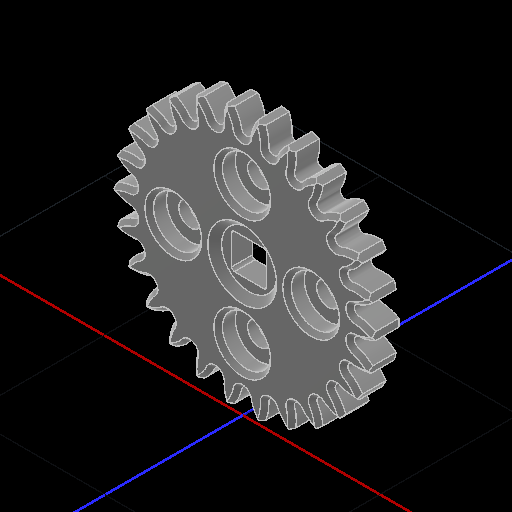
# Autodesk Inventor part: 26t
Saved by Autodesk Inventor 2025.2 (Build 292293000, 293)
## iProperties
Created: 2025-11-16
Part Number: 26t
Material: white pla
Document SubType Name: Modeling
Designer: cloudy
Density: 1 g/cm^3
Appearance: Smooth - Dark Gray
Mass: 8.30169 g
Surface Area: 51.1957 cm^2
Volume: 8.30169 cm^3
Author: cloudy
Autodesk Inventor part; units mm, degrees
ref_plane "YZ Plane" through (0, 0, 0) normal (1, 0, 0) x (0, 1, 0)
ref_plane "XZ Plane" through (0, 0, 0) normal (0, 1, 0) x (-1, 0, 0)
ref_plane "XY Plane" through (0, 0, 0) normal (0, 0, 1) x (1, 0, 0)
sketch "Sketch1" plane through (0, 0, 0) normal (0, 0, 1) x (1, 0, 0)
  spline S0 degree 3 poles (-2.1609, 23.7142) (-2.1092, 23.6364) (-2.0057, 23.4806) (-1.8586, 23.2418) (-1.7174, 22.9994) (-1.5833, 22.7529) (-1.4568, 22.5025) (-1.3387, 22.2481) (-1.2298, 21.9896) (-1.1311, 21.7269) (-1.0453, 21.4599) (-0.9712, 21.1889) (-0.9358, 20.9577) (-0.8951, 20.7751) (-0.8519, 20.6415) (-0.7979, 20.5119) (-0.7264, 20.3909) (-0.6401, 20.2798) (-0.5521, 20.2018) (-0.4739, 20.1504) (-0.4118, 20.1177) (-0.347, 20.0908) (-0.2793, 20.0718) (-0.2104, 20.0585) (-0.1169, 20.053) (0, 20.0563) (0.1169, 20.053) (0.2104, 20.0585) (0.2793, 20.0718) (0.347, 20.0908) (0.4118, 20.1177) (0.4739, 20.1504) (0.5521, 20.2018) (0.6401, 20.2798) (0.7264, 20.3909) (0.7979, 20.5119) (0.8519, 20.6415) (0.8951, 20.7751) (0.9358, 20.9577) (0.9712, 21.1889) (1.0453, 21.4599) (1.1311, 21.7269) (1.2298, 21.9896) (1.3387, 22.2481) (1.4568, 22.5025) (1.5833, 22.7529) (1.7174, 22.9994) (1.8586, 23.2418) (2.0057, 23.4806) (2.1092, 23.6364) (2.1609, 23.7142) knots 0 0 0 0 0.028048 0.056097 0.084146 0.112194 0.140242 0.16829 0.196338 0.224386 0.252432 0.280477 0.308521 0.322545 0.336563 0.350579 0.36459 0.378601 0.392611 0.399624 0.406632 0.413644 0.420653 0.427666 0.434674 0.448699 0.462724 0.469733 0.476745 0.483754 0.490767 0.497774 0.504787 0.518798 0.532808 0.546819 0.560835 0.574853 0.588877 0.616922 0.644966 0.673013 0.70106 0.729108 0.757156 0.785204 0.813253 0.841301 0.86935 0.897398 0.897398 0.897398 0.897398
  circle A0 centre (0, 0) radius 20.055 construction
  circle A1 centre (0, 0) radius 20.8847 construction
  circle A2 centre (0, 0) radius 22.225 construction
  circle A3 centre (0, 0) radius 23.8125
  point P0 (-2.0071, 23.4797)
  point P1 (-1.8596, 23.2412)
  point P2 (-1.7186, 22.9987)
  point P3 (-1.5846, 22.7523)
  point P4 (-1.4582, 22.5019)
  point P5 (-1.3402, 22.2474)
  point P6 (-1.2315, 21.9889)
  point P7 (-1.1332, 21.7262)
  point P8 (-1.0472, 21.4592)
  point P9 (-0.9765, 21.1878)
  point P10 (-0.9246, 20.9122)
  point P11 (-0.893, 20.7756)
  point P12 (-0.8501, 20.6422)
  point P13 (-0.795, 20.5133)
  point P14 (-0.7239, 20.3925)
  point P15 (-0.6369, 20.2827)
  point P16 (-0.532, 20.1899)
  point P17 (-0.4733, 20.1514)
  point P18 (-0.4114, 20.1187)
  point P19 (-0.3465, 20.0921)
  point P20 (-0.2791, 20.0727)
  point P21 (-0.2102, 20.06)
  point P22 (-0.1402, 20.0551)
  point P23 (0, 20.055)
  point P24 (0.1402, 20.0551)
  point P25 (0.2102, 20.06)
  point P26 (0.2791, 20.0727)
  point P27 (0.3465, 20.0921)
  point P28 (0.4114, 20.1187)
  point P29 (0.4733, 20.1514)
  point P30 (0.532, 20.1899)
  point P31 (0.6369, 20.2827)
  point P32 (0.7239, 20.3925)
  point P33 (0.795, 20.5133)
  point P34 (0.8501, 20.6422)
  point P35 (0.893, 20.7756)
  point P36 (0.9246, 20.9122)
  point P37 (0.9765, 21.1878)
  point P38 (1.0472, 21.4592)
  point P39 (1.1332, 21.7262)
  point P40 (1.2315, 21.9889)
  point P41 (1.3402, 22.2474)
  point P42 (1.4582, 22.5019)
  point P43 (1.5846, 22.7523)
  point P44 (1.7186, 22.9987)
  point P45 (1.8596, 23.2412)
  point P46 (2.0071, 23.4797)
  constraints: 4 centre point, 2 point on circle, 103 other
extrude "Extrusion1" add sketch "Sketch1" against normal blind 5.08
extrude "Extrusion2" cut sketch "Sketch1" against normal through all contours A3 S0 picked at (-0.2752, 22.8019)
chamfer "Chamfer1" distance 0.7937 angle 45 1 edges at (0, 20.055, 0)
pattern_circular "Circular Pattern1" count 26 over 360 about axis through (0, 0, 0) along (0, 0, -1) of "Extrusion2", "Chamfer1"
sketch "Sketch2" plane through (0, 0, 0) normal (0, 0, 1) x (1, 0, 0)
  circle A0 centre (0, 0) radius 2.54
  dimension "d10" = 5.08
  constraints: 1 centre point, 1 coincident
  measures "d10" diameter of A0
extrude "Extrusion3" cut sketch "Sketch2" against normal through all
sketch "Sketch3" plane through (0, 0, 0) normal (0, 0, 1) x (1, 0, 0)
  circle A0 centre (-12.7, 0) radius 2.1844
  line L0 (0, 0) -> (-12.7, 0) construction
  dimension "d13" = 4.3688
  dimension "d14" = 12.7
  constraints: 2 end point, 1 centre point, 1 horizontal
  measures "d13" diameter of A0
  measures "d14" distance of L0.start L0.end
extrude "Extrusion4" cut sketch "Sketch3" against normal through all
sketch "Sketch4" plane through (0, 0, 0) normal (0, 0, 1) x (1, 0, 0)
  circle A0 centre (-12.7, 0) radius 2.1844 projected
  circle A1 centre (-12.7, 0) radius 4.445
  point P0 (0, 0)
  dimension "d17" = 8.89
  constraints: 1 centre point, 1 coincident
  measures "d17" diameter of A1
extrude "Extrusion5" cut sketch "Sketch4" against normal blind 3.175
chamfer "Chamfer2" distance 0.7937 angle 45 1 edges at (-17.145, 0, 0)
sketch "Sketch5" plane through (0, 0, 0) normal (0, 0, 1) x (1, 0, 0)
  circle A0 centre (0, 0) radius 5.08
  dimension "d23" = 10.16
  constraints: 1 centre point, 1 coincident
  measures "d23" diameter of A0
extrude "Extrusion6" cut sketch "Sketch5" against normal blind 1.27
chamfer "Chamfer3" distance 1.27 angle 45 1 edges at (-5.08, 0, 0)
pattern_circular "Circular Pattern2" count 4 over 360 about axis through (0, 0, -0.635) along (0, 0, 1) of "Extrusion5", "Extrusion4", "Chamfer2"
sketch "Sketch6" plane through (0, 0, -1.27) normal (0, 0, 1) x (1, 0, 0)
  line L0 (-3.2258, 3.2258) -> (3.2258, 3.2258)
  line L1 (3.2258, 3.2258) -> (3.2258, -3.2258)
  line L2 (3.2258, -3.2258) -> (-3.2258, -3.2258)
  line L3 (-3.2258, -3.2258) -> (-3.2258, 3.2258)
  circle A0 centre (0, 0) radius 2.54 projected
  line L4 (-3.2258, 3.2258) -> (3.2258, -3.2258) construction
  line L5 (3.2258, 3.2258) -> (-3.2258, -3.2258) construction
  dimension "d32" = 6.4516
  dimension "d33" = 6.4516
  constraints: 12 end point, 2 midpoint, 2 parallel, 1 horizontal, 1 perpendicular
  measures "d32" distance of L1.end L2.end
  measures "d33" distance of L0.end L1.end
extrude "Extrusion7" cut sketch "Sketch6" against normal blind 3.81 contours L0 L1 L2 L3 | A0
fillet "Fillet1" radius 0.508 4 edges at (-3.2258, 3.2258, -3.175) (-3.2258, -3.2258, -3.175) (3.2258, -3.2258, -3.175) (3.2258, 3.2258, -3.175)
equation "\"Module\" = 1.5875"
equation "\"PressureAngle\" = 20deg"
equation "\"UnitProfileClearance\" = 0.25"
equation "\"UnitRoundRadius\" = 0.35"
equation "\"HeadDiameter\" = 47.625"
equation "\"RootDiameter\" = 40.10993"
equation "\"BaseDiameter\" = 41.76934"
equation "\"PitchDiameter\" = 44.45"
equation "\"FaceWidth\" = 6.35"
equation "\"HelixAngle\" = 0"
equation "\"UnitCorrection\" = 0"
equation "\"UnitAddendumModification\" = 0"
equation "\"CircularPitch\" = 4.98728"
equation "\"UnitBacklashShift\" = -0.116952"
equation "\"TotalToolShift\" = -0.18566"
equation "\"IsInternal\" = 0"
body "Solid1"
